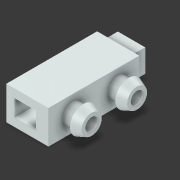
# Autodesk Inventor part: manifold_lower
Saved by Autodesk Inventor 2020.2 (Build 242310000, 310)
## iProperties
Created: 2020-07-06
Part Number: manifold_lower
Material: PLA (Blue-glowing, 3D Printed)
Document SubType Name: Modeling
Designer: isaac
Density: 1 g/cm^3
Appearance: PLA (Blue-glowing)
Author: isaac
Autodesk Inventor part; units mm, degrees
ref_plane "Start Plane" through (-5.7625, 0, 0) normal (1, 0, 0) x (0, 1, 0)
ref_plane "End Plane" through (15.7875, 0, 0) normal (1, 0, 0) x (0, 1, 0)
sketch "Box Sketch" plane through (0, 0, 0) normal (1, 0, 0) x (0, 1, 0)
  line L0 (-3.9688, 0) -> (3.9688, 0)
  line L1 (3.9688, 0) -> (3.9688, 10)
  line L2 (3.9688, 10) -> (-3.9688, 10)
  line L3 (-3.9688, 10) -> (-3.9688, 0)
  line L4 (-1.9688, 2) -> (1.9688, 2)
  line L5 (1.9688, 2) -> (1.9687, 7)
  line L6 (1.9687, 7) -> (-1.9687, 7)
  line L7 (-1.9687, 7) -> (-1.9688, 2)
  line L8 (1.9688, 2) -> (3.9688, 2) construction
  line L9 (-1.9688, 2) -> (-3.9688, 2) construction
  line L10 (-1.9688, 2) -> (-1.9688, 0) construction
  line L11 (2.7188, 1.25) -> (2.7188, 7.75)
  line L12 (2.7188, 7.75) -> (-2.7188, 7.75)
  line L13 (-2.7188, 7.75) -> (-2.7188, 1.25)
  line L14 (-2.7188, 1.25) -> (2.7188, 1.25)
  line L15 (-1.9687, 7) -> (-2.7188, 7) construction
  line L16 (1.9687, 7) -> (2.7188, 7) construction
  line L17 (1.9688, 2) -> (1.9687, 1.25) construction
  line L18 (-1.9687, 7) -> (-1.9687, 7.75) construction
  line L19 (-2.8688, 7.9) -> (2.8688, 7.9)
  line L20 (2.8688, 7.9) -> (2.8688, 1.1)
  line L21 (2.8688, 1.1) -> (-2.8688, 1.1)
  line L22 (-2.8688, 1.1) -> (-2.8688, 7.9)
  point P0 (0, 0)
  point P1 (0, 0)
  dimension "boxHeight" = 7.9375
  dimension "boxWidth" = 10
  dimension "frontWallThick" = 3
  dimension "sideWallThick" = 2
  dimension "connectorTol" = 0.15
  dimension "d24" = 0.75
  constraints: 46 end point, 9 point on line, 6 horizontal, 5 equal length, 5 vertical, 4 parallel, 2 perpendicular, 1 coincident, 1 midpoint, 3 other
  measures "boxHeight" distance of L2.end L1.end
  measures "boxWidth" distance of L1.end L0.end
  measures "frontWallThick" distance between parallel lines of L2 L6
  measures "sideWallThick" distance between parallel lines of L0 L4
  measures "connectorTol" distance between parallel lines of L12 L19
  measures "d24" distance between parallel lines of L4 L14
sketch "Fitting Sketch" plane through (0, 0, 0) normal (1, 0, 0) x (0, 1, 0)
  line L0 (0, 10) -> (0, 14.5) construction
  line L1 (2.3813, 10) -> (2.3813, 12.0417)
  line L2 (2.3813, 12.0417) -> (3.175, 12.5)
  line L3 (3.175, 12.5) -> (2.3813, 14.5)
  line L4 (2.3813, 14.5) -> (1.5, 14.5)
  line L5 (1.5, 14.5) -> (1.5, 10)
  line L6 (1.5, 10) -> (2.3813, 10)
  point P0 (0, 0)
  dimension "d2" = 3
  dimension "d3" = 2
  dimension "d4" = 60
  dimension "d5" = 2.5
  dimension "d6" = 4.7625
  dimension "d7" = 6.35
  dimension "d9" = 10
  constraints: 14 end point, 4 point on line, 3 vertical, 2 horizontal
  measures "d2" diameter of L5 L0
  measures "d3" vertical distance of L2.end L3.end
  measures "d4" angle of L1 L2
  measures "d5" distance from line of L6 L2.end
  measures "d6" diameter of L1 L0
  measures "d7" diameter of L2.end L0
  measures "d9" distance of point (0, 0) L0.start
revolve "Fitting" add sketch "Fitting Sketch" angle 360 about axis through (0, 0, 10) along (0, 0, 1)
extrude "Box" add sketch "Box Sketch" along normal mid plane 11.525 contours L3 L2 L1 L0 | L14 L13 L12 L11 | L19 L20 L21 L22
ref_plane "Loft Start Plane" through (0, 0, 7) normal (0, 0, 1) x (1, 0, 0)
sketch "Loft Sketch" plane through (0, 0, 7) normal (0, 0, 1) x (1, 0, 0)
  line L0 (1.5, -1.9688) -> (-1.5, -1.9688)
  line L1 (-1.5, -1.9688) -> (-1.5, 1.9687)
  line L2 (-1.5, 1.9687) -> (1.5, 1.9687)
  line L3 (1.5, 1.9687) -> (1.5, -1.9688)
  line L4 (1.5, -1.9688) -> (-1.5, 1.9687) construction
  line L5 (-1.5, -1.9688) -> (1.5, 1.9687) construction
  point P0 (0, 0)
  dimension "d17" = 3
  dimension "d18" = 3.9375
  constraints: 12 end point, 2 midpoint, 2 parallel, 1 horizontal, 1 perpendicular
  measures "d17" distance of L1.end L2.end
  measures "d18" distance of L0.end L1.end
loft "Loft" cut profiles "Loft Sketch" section 1 edges at (0, -1.5, 10)
pattern_linear "Channel Repetition" count 2 spacing 10.775 along (1, 0, 0)
extrude "Clip Extra Length" cut sketch "Box Sketch" along normal blind 19.45 from surface at 15.7875 contours L3 L2 L1 L0 | L19 L20 L21 L22
extrude "Connector" add sketch "Box Sketch" along normal blind 3.6625 from surface at 15.7875 contours L14 L13 L12 L11
equation "\"boxHeight\" = fittingBarbOD + 2 * siliconeThick"
equation "\"boxWidth\" = manifoldWidth"
equation "\"d2\" = fittingID"
equation "\"d3\" = fittingBarbLength"
equation "\"d4\" = fittingBarbBaseAngle"
equation "\"d5\" = fittingNeckLength"
equation "\"d6\" = fittingOD"
equation "\"d7\" = fittingBarbOD"
equation "\"d9\" = boxWidth"
equation "\"d14\" = blockWidth"
equation "\"d27\" = chanWidth"
equation "\"d17\" = fittingID"
equation "\"d18\" = boxHeight - 2 * sideWallThick"
equation "\"d16\" = boxWidth - frontWallThick"
equation "\"d29\" = -0.5 * blockWidth"
equation "\"fittingBarbOD\" = 6.35"
equation "\"siliconeThick\" = 0.79375"
equation "\"manifoldWidth\" = 10"
equation "\"fittingID\" = 3"
equation "\"fittingBarbLength\" = 2"
equation "\"fittingBarbBaseAngle\" = 60deg"
equation "\"fittingNeckLength\" = 2.5"
equation "\"fittingOD\" = 4.7625"
equation "\"blockWidth\" = 11.525"
equation "\"chanWidth\" = 10.775"
body "Solid1"
